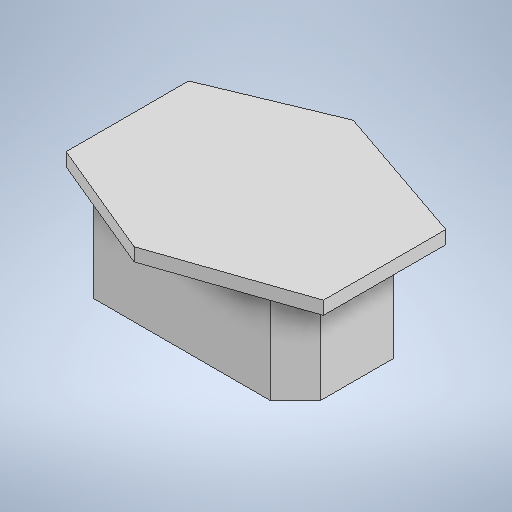
# Autodesk Inventor part: power_test
Saved by Autodesk Inventor 2025 (Build 290162000, 162)
## iProperties
Created: 2024-12-15
Part Number: power_test
Material: Generic
Document SubType Name: Modeling
Designer: ethan
Density: 1 g/cm^3
Appearance: Default
Author: ethan
Autodesk Inventor part; units mm, degrees
ref_plane "YZ Plane" through (0, 0, 0) normal (1, 0, 0) x (0, 1, 0)
ref_plane "XZ Plane" through (0, 0, 0) normal (0, 1, 0) x (-1, 0, 0)
ref_plane "XY Plane" through (0, 0, 0) normal (0, 0, 1) x (1, 0, 0)
sketch "Sketch1" plane through (0, 0, 0) normal (0, 1, 0) x (-1, 0, 0)
  line L0 (5.6569, 0) -> (36, 0)
  line L1 (36, -28) -> (5.6569, -28)
  line L2 (0, -5.6568) -> (5.6569, 0)
  line L3 (36, -14) -> (0, -14) construction
  line L4 (5.6569, -28) -> (36, -28)
  line L5 (0, -22.3432) -> (5.6569, -28)
  line L6 (41, -28) -> (41, 5) construction
  line L7 (41, 5) -> (3.5859, 5) construction
  line L8 (3.5859, 5) -> (-3.5355, -2.1212) construction
  line L9 (36, -33) -> (5.6569, -33) construction
  line L10 (36, 0) -> (46, 0) construction
  line L11 (46, 0) -> (46, -28) construction
  line L12 (46, -28) -> (36, -28) construction
  line L13 (36, -28) -> (36, 0) construction
  line L14 (51, 5) -> (31, 5) construction
  line L15 (31, 5) -> (31, -33) construction
  line L16 (31, -33) -> (51, -33) construction
  line L17 (51, -33) -> (51, 5) construction
  line L18 (0, 0) -> (-5, 0) construction
  line L19 (-5, 0) -> (-5, -8.8109) construction
  line L20 (-5, -8.8109) -> (0, -8.8109) construction
  line L21 (0, -8.8109) -> (0, 0) construction
  line L22 (36, 0) -> (46, 0)
  line L23 (46, 0) -> (46, -28)
  line L24 (46, -28) -> (36, -28)
  line L25 (0, -5.6568) -> (0, -22.3432)
  dimension "d1" = 28
  dimension "d3" = 8
  dimension "d5" = 5
  dimension "d6" = 10
  dimension "d7" = 5
  dimension "d8" = 5
  constraints: 52 end point, 9 parallel, 5 perpendicular, 4 horizontal, 2 symmetric about line, 1 collinear, 4 other
  measures "d1" distance of L0.end L1.start
  measures "d3" distance of L0.start L2.start
  measures "d5" distance between parallel lines of L1 L9
  measures "d6" distance of L11.end L12.end
  measures "d7" distance between parallel lines of L10 L14
  measures "d8" distance of L20.end L19.end
extrude "Extrusion1" add sketch "Sketch1" along normal blind 22.86
sketch "Sketch2" plane through (0, 22.86, 0) normal (0, 1, 0) x (1, 0, 0)
  line L0 (-46, 28) -> (-46, 0) construction
  line L1 (-46, 0) -> (-5.6569, 0) construction
  line L2 (-5.6569, 0) -> (0, 5.6568) construction
  line L3 (0, 5.6568) -> (0, 22.3432) construction
  line L4 (0, 22.3432) -> (-5.6569, 28) construction
  line L5 (-5.6569, 28) -> (-46, 28) construction
  line L6 (-46, 14) -> (-52.35, 14) construction
  line L7 (0, 14) -> (6.35, 14) construction
  line L8 (-25.8285, 28) -> (-25.8285, 39) construction
  line L9 (-46, 0) -> (-5.6569, 0) construction
  line L10 (-25.8285, 0) -> (-25.8285, -11) construction
  line L11 (-52.35, 14) -> (-52.35, 27.97) construction
  line L12 (-52.35, 27.97) -> (-52.35, 0.03) construction
  line L13 (6.35, 14) -> (6.35, 27.97) construction
  line L14 (6.35, 27.97) -> (6.35, 0.03) construction
  line L15 (-52.35, 0.03) -> (-25.8285, -11)
  line L16 (-25.8285, -11) -> (6.35, 0.03)
  line L17 (6.35, 0.03) -> (6.35, 27.97)
  line L18 (6.35, 27.97) -> (-25.8285, 39)
  line L19 (-25.8285, 39) -> (-52.35, 27.97)
  line L20 (-52.35, 0.03) -> (-52.35, 27.97)
  point P0 (0, 0)
  dimension "d11" = 6.35
  dimension "d12" = 6.35
  dimension "d13" = 11
  dimension "d14" = 11
  dimension "d15" = 13.97
  dimension "d16" = 27.94
  dimension "d17" = 13.97
  dimension "d18" = 27.94
  constraints: 28 end point, 4 midpoint, 4 vertical, 2 collinear, 2 horizontal, 2 point on line
  measures "d11" distance of L6.start L6.end
  measures "d12" distance of L7.start L7.end
  measures "d13" distance of L8.start L8.end
  measures "d14" distance of L10.start L10.end
  measures "d15" distance of L6.end L11.end
  measures "d16" distance of L11.end L12.end
  measures "d17" distance of L7.end L13.end
  measures "d18" distance of L13.end L14.end
extrude "Extrusion2" add sketch "Sketch2" along normal blind 3
body "Solid1"
